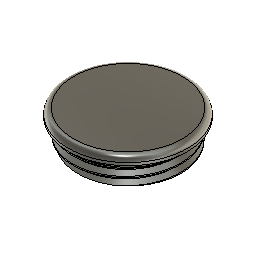
projectdoosje dopje v1 (Autodesk Fusion 360 design; units mm, degrees)
Autodesk Fusion 360 part; units mm, degrees
sketch "Sketch1" plane through (0, 0, 0) normal (0, 0, 1) x (1, 0, 0)
  circle A0 centre (0, 0) radius 10
  dimension "d1" = 20
  constraint coincident A0.centre origin
  measures "d1" diameter of A0
extrude "Extrude1" add sketch "Sketch1" along normal blind 5
sketch "Sketch2" plane through (0, 0, 5) normal (0, 0, 1) x (-1, 0, 0)
  circle A0 centre (0, 0) radius 10
  circle A1 centre (0, 0) radius 11
  dimension "d4" = 22
  constraint coincident A0.centre A1.centre
  measures "d4" diameter of A1
extrude "Extrude2" add sketch "Sketch2" along normal blind 1.5 contours A0 | A1
fillet "Fillet1" radius 1 1 edges at (10.2556, 3.9778, 6.5)
thread "Thread1" "ISO Metric profile 20.0 M20x1.5 6g" major diameter 19.85 minor diameter 18.137 pitch 1.5 angle 60 modelled right hand crest width 0.2154 on face at (9.9876, -0.4985, 3.3333) from (0, 0, 0) to (0, 0, 4) crest through (9.925, 0, -0.375)
sketch "Sketch3" plane through (0, 0, 0) normal (0, 1, 0) x (1, 0, 0)
  line L0 (-10, -4) -> (-9, -4)
  line L1 (-9, -4) -> (-9, -5)
  line L2 (-9, -5) -> (-10, -5)
  line L3 (-10, -5) -> (-10, -4)
  line L4 (0, 0) -> (0, -8.306) construction
  line L5 (-9, -1.0283) -> (-7, 1)
  line L6 (-7, 1) -> (-10, 1)
  line L7 (-10, 1) -> (-10, -1)
  line L8 (-10, -1) -> (-9, -1.0283)
  dimension "d11" = 9
  dimension "d12" = 10
  dimension "d14" = 9
  dimension "d15" = 10
  constraint horizontal L0
  constraint vertical L1
  constraint horizontal L2
  constraint vertical L3
  constraint coincident L4.start origin
  constraint vertical L4
  constraint perpendicular L1 L6
  constraint perpendicular L0 L7
  measures "d11" distance of L1 L4
  measures "d12" distance of L3 L4
  measures "d14" distance of L4 L5.start
  measures "d15" distance of L4.start L7
revolve "Revolve1" cut sketch "Sketch3" angle 360 about axis through (0, 0, 0) along (0, 0, -1)
equation "d14 = d11"
